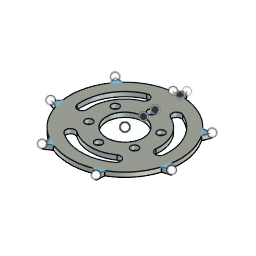
48mm Cleat 7Spikes (Autodesk Fusion 360 design; units mm, degrees)
Autodesk Fusion 360 part; units mm, degrees
sketch "Sketch1" plane through (0, 0, 0) normal (0, 0, 1) x (1, 0, 0)
  circle A0 centre (0, 0) radius 24
  circle A1 centre (0, 0) radius 11.5
  line L0 (0, 0) -> (0, 11.5)
  line L1 (0, 0) -> (-9.9593, 5.75)
  line L2 (0, 0) -> (9.9593, 5.75)
  line L3 (0, 0) -> (9.9593, -5.75)
  line L4 (0, 0) -> (0, -11.5)
  line L5 (0, 0) -> (-9.9593, -5.75)
  circle A2 centre (0, 11.5) radius 1.6
  circle A3 centre (9.9593, 5.75) radius 1.6
  circle A4 centre (9.9593, -5.75) radius 1.6
  circle A5 centre (0, -11.5) radius 1.6
  circle A6 centre (-9.9593, -5.75) radius 1.6
  circle A7 centre (-9.9593, 5.75) radius 1.6
  line L6 (0, 11.5) -> (-5, 11.5)
  line L7 (0, 11.5) -> (5, 11.5)
  line L8 (9.9593, -5.75) -> (7.4593, -10.0801)
  line L9 (9.9593, -5.75) -> (12.4593, -1.4199)
  line L10 (-9.9593, -5.75) -> (-7.4593, -10.0801)
  line L11 (-9.9593, -5.75) -> (-12.4593, -1.4199)
  circle A8 centre (0, 0) radius 19
  line L12 (-5, 11.5) -> (-5, 10.3562)
  line L13 (5, 11.5) -> (5, 10.3562)
  line L14 (12.4593, -1.4199) -> (11.4687, -0.848)
  line L15 (7.4593, -10.0801) -> (6.4687, -9.5082)
  line L16 (-7.4593, -10.0801) -> (-6.4687, -9.5082)
  line L17 (-12.4593, -1.4199) -> (-11.4687, -0.848)
  line L18 (-12.4593, -1.4199) -> (-18.3745, -4.835)
  line L19 (-7.4593, -10.0801) -> (-13.3745, -13.4953)
  line L20 (7.4593, -10.0801) -> (13.3745, -13.4953)
  line L21 (12.4593, -1.4199) -> (18.3745, -4.835)
  line L22 (5, 11.5) -> (5, 18.3303)
  line L23 (-5, 11.5) -> (-5, 18.3303)
  circle A9 centre (0, 0) radius 8
  circle A10 centre (0, 0) radius 15
  line L24 (0, 24) -> (-15.4269, 18.3851)
  line L25 (-15.4269, 18.3851) -> (-23.6354, 4.1676)
  line L26 (-23.6354, 4.1676) -> (-20.7846, -12)
  line L27 (-20.7846, -12) -> (-8.2085, -22.5526)
  line L28 (-8.2085, -22.5526) -> (8.2085, -22.5526)
  line L29 (8.2085, -22.5526) -> (20.7846, -12)
  line L30 (20.7846, -12) -> (23.6354, 4.1676)
  line L31 (23.6354, 4.1676) -> (15.4269, 18.3851)
  line L32 (15.4269, 18.3851) -> (0, 24)
  line L33 (0, 24) -> (0.2615, 26.9886)
  line L34 (0, 24) -> (3, 24) construction
  line L35 (0.2615, 26.9886) -> (-1.883, 23.926)
  line L36 (0.2615, 26.9886) -> (4.0002, 26.9886) construction
  dimension "d1" = 48
  dimension "d2" = 23
  dimension "d3" = 3.2
  dimension "d4" = 3.2
  dimension "d5" = 3.2
  dimension "d6" = 3.2
  dimension "d7" = 3.2
  dimension "d8" = 3.2
  dimension "d9" = 5
  dimension "d10" = 5
  dimension "d11" = 5
  dimension "d12" = 5
  dimension "d13" = 5
  dimension "d14" = 38
  dimension "d15" = 16
  dimension "d16" = 30
  dimension "d17" = 85
  dimension "d18" = 3
  dimension "d19" = 125
  constraint coincident A0.centre A1.centre
  constraint concentric A0 A1
  constraint coincident A1 L0.end
  constraint vertical L0
  constraint coincident A1 L1.end
  constraint coincident A1 L2.end
  constraint coincident A1 L3.end
  constraint parallel L1 L3
  constraint coincident A1 L4.end
  constraint parallel L0 L4
  constraint coincident A1 L5.end
  constraint parallel L2 L5
  constraint coincident L0.end A2.centre
  constraint coincident L2.end A3.centre
  constraint coincident L3.end A4.centre
  constraint coincident L4.end A5.centre
  constraint coincident L5.end A6.centre
  constraint coincident L1.end A7.centre
  constraint perpendicular L0 L6
  constraint perpendicular L0 L7
  constraint perpendicular L3 L8
  constraint perpendicular L3 L9
  constraint tangent A1 L10
  constraint perpendicular L5 L10
  constraint perpendicular L5 L11
  constraint concentric A0 A8
  constraint coincident A1 L12.end
  constraint vertical L12
  constraint coincident A1 L13.end
  constraint perpendicular L7 L13
  constraint coincident A1 L14.end
  constraint perpendicular L9 L14
  constraint coincident A1 L15.end
  constraint perpendicular L8 L15
  constraint coincident A1 L16.end
  constraint perpendicular L10 L16
  constraint coincident A1 L17.end
  constraint perpendicular L11 L17
  constraint coincident A8 L18.end
  constraint perpendicular L11 L18
  constraint coincident A8 L19.end
  constraint perpendicular L10 L19
  constraint coincident A8 L20.end
  constraint perpendicular L8 L20
  constraint coincident A8 L21.end
  constraint perpendicular L9 L21
  constraint coincident A8 L22.end
  constraint perpendicular L7 L22
  constraint coincident A8 L23.end
  constraint perpendicular L6 L23
  constraint concentric A8 A9
  constraint concentric A8 A10
  constraint coincident A0 L24.start
  constraint horizontal L34
  constraint horizontal L36
  constraint coincident A0 L35.end
  measures "d1" diameter of A0
  measures "d2" diameter of A1
  measures "d3" diameter of A2
  measures "d4" diameter of A3
  measures "d5" diameter of A4
  measures "d6" diameter of A5
  measures "d7" diameter of A6
  measures "d8" diameter of A7
  measures "d9" distance of L0.end L6.end
  measures "d10" distance of L0.end L7.end
  measures "d11" distance of L3.end L8.end
  measures "d12" distance of L3.end L9.end
  measures "d13" distance of L5.end L11.end
  measures "d14" diameter of A8
  measures "d15" diameter of A9
  measures "d16" diameter of A10
  measures "d17" angle of L33 L34
  measures "d18" distance of L24.start L33.end
  measures "d19" angle of L35 L36
extrude "Extrude1" add sketch "Sketch1" along normal blind 2 contours A0 L30 | A0 L31 | L24 L25 L26 L27 L28 L29 L30 L31 L32 | A0 L29 | A0 L32 | A0 L28 | A0 L24 | A0 L27 | A0 L25 | A0 L26 | A1 L2 L3 A3 A4 A9 | A1 A4 L9 L14 | A1 A3 L13 L14 L21 L22 A10 | A4 L8 L9 L20 L21 A10 | A1 L3 L4 A4 A5 A9 | A8 L20 L21 A10 | A1 L0 L2 A2 A3 A9 | A1 A4 L8 L15 | A1 A5 L15 L16 L19 L20 A10 | A1 L4 L5 A5 A6 A9 | A6 L10 L11 L18 L19 A10 | A8 L18 L19 A10 | A8 L22 L23 A10 | A2 L6 L7 L22 L23 A10 | A1 A2 L7 L13 | A1 L0 L1 A2 A7 A9 | A1 L1 L5 A6 A7 A9 | A1 A6 L10 L16 | A1 A7 L12 L17 L18 L23 A10 | A1 A6 L11 L17 | A1 A2 L6 L12
fillet "Fillet1" radius 2 12 edges at (5, 18.3303, 1) (5, 14.1421, 1) (14.7474, -2.7409, 1) (18.3745, -4.835, 1) (13.3745, -13.4953, 1) (9.7474, -11.4012, 1) (-9.7474, -11.4012, 1) (-13.3745, -13.4953, 1) (-18.3745, -4.835, 1) (-14.7474, -2.7409, 1) (-5, 14.1421, 1) (-5, 18.3303, 1)
sketch "Sketch2" plane through (0, 0, 2) normal (0, 0, 1) x (-1, 0, 0)
  circle A0 centre (9.9593, 5.75) radius 1.6
  circle A1 centre (0, 0) radius 8
  circle A2 centre (0, -11.5) radius 1.6
  arc A3 (8.7498, 12.1837) -> (11.083, 15.4326) centre (9.9164, 13.8081) ccw
  arc A4 (8.7498, 12.1837) -> (-8.7498, 12.1837) centre (0, 0) ccw
  arc A5 (-11.083, 15.4326) -> (-8.7498, 12.1837) centre (-9.9164, 13.8081) ccw
  arc A6 (11.083, 15.4326) -> (-11.083, 15.4326) centre (0, 0) ccw
  circle A7 centre (9.9593, -5.75) radius 1.6
  arc A8 (6.1765, -13.6694) -> (7.8235, -17.3145) centre (7, -15.4919) ccw
  arc A9 (6.1765, -13.6694) -> (14.9262, 1.4857) centre (0, 0) ccw
  arc A10 (18.9066, 1.8819) -> (14.9262, 1.4857) centre (16.9164, 1.6838) ccw
  arc A11 (7.8235, -17.3145) -> (18.9066, 1.8819) centre (0, 0) ccw
  arc A12 (-18.9066, 1.8819) -> (-7.8235, -17.3145) centre (0, 0) ccw
  arc A13 (-14.9262, 1.4857) -> (-18.9066, 1.8819) centre (-16.9164, 1.6838) ccw
  arc A14 (-14.9262, 1.4857) -> (-6.1765, -13.6694) centre (0, 0) ccw
  arc A15 (-7.8235, -17.3145) -> (-6.1765, -13.6694) centre (-7, -15.4919) ccw
  circle A16 centre (-9.9593, -5.75) radius 1.6
  circle A17 centre (0, 11.5) radius 1.6
  circle A18 centre (-9.9593, 5.75) radius 1.6
  circle A19 centre (0, 0) radius 24
  line L0 (0, -8) -> (0, -13.1)
  line L1 (0, -24) -> (3.0935, -24) construction
  line L2 (0, -24) -> (0, -27)
  line L3 (0, -24) -> (3.0102, -24) construction
  line L4 (0, -27) -> (1.7698, -23.9347)
  line L5 (0, -27) -> (-1.7698, -23.9347)
  arc A20 (0, -27) -> (0, -27) centre (0, 0) ccw
  arc A21 (-1.7698, -23.9347) -> (1.7698, -23.9347) centre (0, 0) ccw
  line L6 (21.1095, -16.8342) -> (19.8163, -13.5393)
  line L7 (21.1095, -16.8342) -> (17.6094, -16.3067)
  arc A22 (17.6094, -16.3067) -> (19.8163, -13.5393) centre (0, 0) ccw
  line L8 (26.3231, 6.0081) -> (22.9408, 7.0514)
  line L9 (26.3231, 6.0081) -> (23.7284, 3.6006)
  arc A23 (23.7284, 3.6006) -> (22.9408, 7.0514) centre (0, 0) ccw
  line L10 (11.7149, 24.3262) -> (8.7903, 22.3323)
  line L11 (11.7149, 24.3262) -> (11.9794, 20.7965)
  arc A24 (11.9794, 20.7965) -> (8.7903, 22.3323) centre (0, 0) ccw
  line L12 (-11.7149, 24.3262) -> (-11.9794, 20.7965)
  line L13 (-11.7149, 24.3262) -> (-8.7903, 22.3323)
  arc A25 (-8.7903, 22.3323) -> (-11.9794, 20.7965) centre (0, 0) ccw
  line L14 (-26.3231, 6.0081) -> (-23.7284, 3.6006)
  line L15 (-26.3231, 6.0081) -> (-22.9408, 7.0514)
  arc A26 (-22.9408, 7.0514) -> (-23.7284, 3.6006) centre (0, 0) ccw
  line L16 (-21.1095, -16.8342) -> (-17.6094, -16.3067)
  line L17 (-21.1095, -16.8342) -> (-19.8163, -13.5393)
  arc A27 (-19.8163, -13.5393) -> (-17.6094, -16.3067) centre (0, 0) ccw
  dimension "d24" = 54
  dimension "d30" = 30
  dimension "d46" = 360
  constraint coincident A19 L1.start
  constraint vertical L0
  constraint coincident L1.start A21
  constraint concentric A20 A21
  constraint horizontal L1
  constraint horizontal L3
  constraint vertical L2
  constraint symmetric L2 L4.end L5.end
  constraint symmetric L2 L4.start L5.start
  constraint coincident A1 L0.start
  constraint coincident A2 L0.end
  measures "d24" diameter of A20
  measures "d30" angle of L2 L4
extrude "Extrude5" add sketch "Sketch2" against normal blind 2 contours A19 L8 L9 A23 | A19 L6 L7 A22 | A19 L10 L11 A24 | A19 L2 L4 A21 | A19 L2 L5 A21 | A19 L12 L13 A25 | A19 L16 L17 A27 | A19 L14 L15 A26
